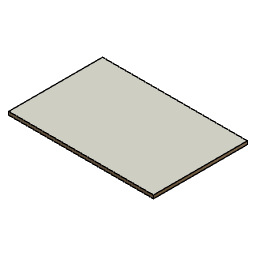
base_plate (Autodesk Fusion 360 design; units mm, degrees)
Autodesk Fusion 360 part; units mm, degrees
sketch "Base Plate" plane through (0, 0, 0) normal (0, 0, 1) x (1, 0, 0)
  line L0 (0, 0) -> (270, 0)
  line L1 (270, 0) -> (270, 175)
  line L2 (270, 175) -> (0, 175)
  line L3 (0, 175) -> (0, 0)
  dimension "d6" = 270
  dimension "d9" = 175
  constraint horizontal L0
  constraint vertical L1
  constraint horizontal L2
  constraint vertical L3
  constraint coincident L0.start L3.end
  measures "d6" distance of L0.start L0.end
  measures "d9" distance of L0.end L1.end
extrude "Extrude1" add sketch "Base Plate" along normal blind 6
equation "MDFThickness = 6 mm" comment "Thickness of the MDF board"
equation "d2 = MDFThickness"
equation "d9 = sidePanelDepth - 2 * clearance"
equation "clearance = 10 mm" comment "Clearance between side panel edge and main body edge"
equation "sidePanelDepth = 195 mm" comment "Depth of the side panel"
named bodies: "Base Plate"
